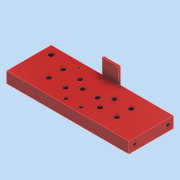
# Autodesk Inventor part: universal_mount
Saved by Autodesk Inventor 2022 (Build 260153000, 153)
## iProperties
Created: 2021-04-19
Part Number: universal_mount
Material: Generic
Document SubType Name: Modeling
Designer: nnico
Density: 1 g/cm^3
Appearance: Red
Author: nnico
Autodesk Inventor part; units mm, degrees
ref_plane "YZ Plane" through (0, 0, 0) normal (1, 0, 0) x (0, 1, 0)
ref_plane "XZ Plane" through (0, 0, 0) normal (0, 1, 0) x (-1, 0, 0)
ref_plane "XY Plane" through (0, 0, 0) normal (0, 0, 1) x (1, 0, 0)
sketch "Sketch1" plane through (0, 0, 0) normal (0, 1, 0) x (-1, 0, 0)
  line L0 (110, -40) -> (-110, -40)
  line L1 (-110, -40) -> (-110, 40)
  line L2 (-110, 40) -> (110, 40)
  line L3 (110, 40) -> (110, -40)
  line L4 (0, -40) -> (0, 40) construction
  line L5 (110, 0) -> (-110, 0) construction
  circle A0 centre (13.5, 0) radius 2.5
  circle A1 centre (-13.5, 0) radius 2.5
  line L6 (46, -40) -> (46, 40) construction
  line L7 (61.25, -13) -> (30.75, -13) construction
  line L8 (30.75, -13) -> (30.75, 13) construction
  line L9 (30.75, 13) -> (61.25, 13) construction
  line L10 (61.25, 13) -> (61.25, -13) construction
  line L11 (46, 13) -> (46, -13) construction
  line L12 (61.25, 0) -> (30.75, 0) construction
  circle A2 centre (30.75, -13) radius 2.75
  circle A3 centre (61.25, -13) radius 2.75
  circle A4 centre (61.25, 13) radius 2.75
  circle A5 centre (30.75, 13) radius 2.75
  circle A6 centre (-30.75, -13) radius 2.75
  circle A7 centre (-61.25, -13) radius 2.75
  circle A8 centre (-61.25, 13) radius 2.75
  circle A9 centre (-30.75, 13) radius 2.75
  circle A10 centre (95, -25) radius 5
  circle A11 centre (13.5, 30) radius 1.6
  circle A12 centre (-13.5, 30) radius 1.6
  point P0 (0, 0)
  point P1 (0, 0)
  dimension "d0" = 220
  dimension "d1" = 80
  dimension "d2" = 5
  dimension "d3" = 27
  dimension "d4" = 92
  dimension "d5" = 30.5
  dimension "d6" = 26
  dimension "d7" = 5.5
  dimension "d8" = 5.5
  dimension "d9" = 5.5
  dimension "d10" = 5.5
  dimension "d19" = 10
  dimension "d20" = 15
  dimension "d21" = 3.2
  dimension "d22" = 27
  dimension "d23" = 10
  dimension "d44" = 15
  constraints: 26 end point, 13 centre point, 9 midpoint, 6 symmetric about line, 5 coincident, 4 parallel, 3 perpendicular, 3 point on line, 2 collinear, 2 horizontal, 6 other
  measures "d0" distance of L0.start L0.end
  measures "d1" distance of L2.end L0.start
  measures "d2" diameter of A0
  measures "d3" diameter of A0.centre L4
  measures "d4" diameter of L6 L4
  measures "d5" distance of L8.end L9.end
  measures "d6" distance of L7.end L8.end
  measures "d7" diameter of A2
  measures "d8" diameter of A3
  measures "d9" diameter of A4
  measures "d10" diameter of A5
  measures "d19" diameter of A10
  measures "d20" distance from line of L0 A10.centre
  measures "d21" diameter of A11
  measures "d22" diameter of A11.centre L4
  measures "d23" distance from line of L2 A11.centre
  measures "d44" distance from line of L3 A10.centre
extrude "Extrusion1" add sketch "Sketch1" along normal blind 20
sketch "Sketch2" plane through (0, 20, 0) normal (0, 1, 0) x (1, 0, 0)
  line L0 (110, 40) -> (-110, 40) projected
  line L1 (-15, 40) -> (15, 40)
  line L2 (15, 40) -> (15, 37)
  line L3 (15, 37) -> (-15, 37)
  line L4 (-15, 37) -> (-15, 40)
  line L5 (0, 37) -> (0, 40) construction
  line L6 (-110, -40) -> (110, -40) construction
  line L7 (0, -40) -> (0, 40) construction
  point P0 (0, 0)
  point P1 (15, 40)
  dimension "d26" = 30
  dimension "d27" = 3
  constraints: 12 end point, 4 midpoint, 2 parallel, 2 perpendicular, 1 collinear, 1 horizontal, 1 point on line
  measures "d26" distance of L2.end L3.end
  measures "d27" distance of L1.end L2.end
extrude "Extrusion2" add sketch "Sketch2" along normal blind 30
sketch "Sketch3" plane through (0, 20, 0) normal (0, 1, 0) x (1, 0, 0)
  circle A0 centre (30.75, -13) radius 2.75 projected
  circle A1 centre (61.25, -13) radius 2.75 projected
  circle A2 centre (61.25, 13) radius 2.75 projected
  circle A3 centre (30.75, 13) radius 2.75 projected
  circle A4 centre (13.5, 0) radius 2.5 projected
  circle A5 centre (13.5, -30) radius 1.6 projected
  line L0 (-110, -40) -> (110, -40) construction
  line L1 (0, -40) -> (0, 40) construction
  line L2 (110, 40) -> (-110, 40) construction
  circle A6 centre (13.5, -30) radius 1.6 projected
  circle A7 centre (13.5, -30) radius 3.5
  circle A8 centre (13.5, 0) radius 4.5
  circle A9 centre (30.75, -13) radius 4.5
  circle A10 centre (30.75, 13) radius 4.5
  circle A11 centre (61.25, -13) radius 4.5
  circle A12 centre (61.25, 13) radius 4.5
  circle A13 centre (-30.75, -13) radius 2.75
  circle A14 centre (-61.25, -13) radius 2.75
  circle A15 centre (-61.25, 13) radius 2.75
  circle A16 centre (-30.75, 13) radius 2.75
  circle A17 centre (-13.5, 0) radius 2.5
  circle A18 centre (-13.5, -30) radius 1.6
  circle A19 centre (-13.5, -30) radius 1.6
  circle A20 centre (-13.5, -30) radius 3.5
  circle A21 centre (-13.5, 0) radius 4.5
  circle A22 centre (-30.75, -13) radius 4.5
  circle A23 centre (-30.75, 13) radius 4.5
  circle A24 centre (-61.25, -13) radius 4.5
  circle A25 centre (-61.25, 13) radius 4.5
  point P0 (0, 0)
  dimension "d30" = 7
  dimension "d31" = 9
  dimension "d32" = 9
  dimension "d33" = 9
  dimension "d34" = 9
  dimension "d35" = 9
  constraints: 19 centre point, 13 symmetric about line, 12 coincident, 2 end point, 2 midpoint, 13 other
  measures "d30" diameter of A7
  measures "d31" diameter of A8
  measures "d32" diameter of A9
  measures "d33" diameter of A10
  measures "d34" diameter of A11
  measures "d35" diameter of A12
extrude "Extrusion3" cut sketch "Sketch3" against normal blind 10 contours A3 | A5 | A7 | A8 | A9 | A10 | A11 | A12 | A15 | A18 | A20 | A21 | A22 | A23 | A24 | A25
sketch "Sketch4" plane through (110, 0, 40) normal (1, 0, 0) x (0, 0, -1)
  line L0 (0, 0) -> (0, 20) construction
  line L1 (0, 10) -> (80, 10) construction
  line L2 (80, 0) -> (80, 20) construction
  line L3 (40, 0) -> (40, 20) construction
  line L4 (0, 20) -> (80, 20) construction
  circle A0 centre (10, 10) radius 3.5
  circle A1 centre (70, 10) radius 3.5
  dimension "d38" = 7
  dimension "d39" = 60
  constraints: 4 end point, 3 midpoint, 2 centre point, 1 point on line, 1 symmetric about line, 1 other
  measures "d38" diameter of A0
  measures "d39" diameter of A0.centre L3
extrude "Extrusion4" cut sketch "Sketch4" against normal blind 11
sketch "Sketch5" plane through (-110, 0, -40) normal (-1, 0, 0) x (0, 0, 1)
  circle A0 centre (70, 10) radius 3.5 projected
  circle A1 centre (10, 10) radius 3.5 projected
  point P0 (40, 0)
extrude "Extrusion5" cut sketch "Sketch5" against normal blind 11
sketch "Sketch6" plane through (0, 20, 0) normal (0, 1, 0) x (1, 0, 0)
  circle A0 centre (-50, 30) radius 2.5
  line L0 (15, 40) -> (-15, 40) projected
  line L1 (0, 40) -> (0, 37) construction
  line L2 (15, 37) -> (-15, 37) construction
  point P0 (0, 0)
  dimension "d45" = 5
  dimension "d46" = 10
  dimension "d47" = 50
  constraints: 2 end point, 2 midpoint, 1 centre point
  measures "d45" diameter of A0
  measures "d46" distance from line of L0 A0.centre
  measures "d47" distance from line of L1 A0.centre
extrude "Extrusion6" cut sketch "Sketch6" against normal blind 5
body "Solid1"
